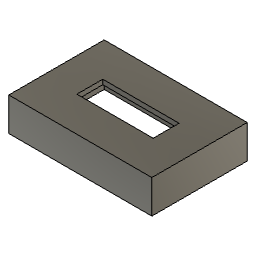
Earpiece (Autodesk Fusion 360 design; units mm, degrees)
Autodesk Fusion 360 part; units mm, degrees
sketch "Esboço1" plane through (0, 0, 0) normal (0, 0, 1) x (1, 0, 0)
  line L0 (75, 50) -> (-75, 50)
  line L1 (-75, 50) -> (-75, -50)
  line L2 (-75, -50) -> (75, -50)
  line L3 (75, -50) -> (75, 50)
  line L4 (75, 50) -> (-75, -50) construction
  line L5 (-75, 50) -> (75, -50) construction
  line L6 (-65, 40) -> (65, 40)
  line L7 (65, 40) -> (65, -40.4734)
  line L8 (65, -40.4734) -> (-65, -40.4734)
  line L9 (-65, -40.4734) -> (-65, 40)
  line L10 (39.9847, -13.5797) -> (-39.9847, -13.5797)
  line L11 (-39.9847, -13.5797) -> (-39.9847, 13.5797)
  line L12 (-39.9847, 13.5797) -> (39.9847, 13.5797)
  line L13 (39.9847, 13.5797) -> (39.9847, -13.5797)
  line L14 (39.9847, -13.5797) -> (-39.9847, 13.5797) construction
  line L15 (-39.9847, -13.5797) -> (39.9847, 13.5797) construction
  constraint horizontal L0
  constraint perpendicular L0 L1
  constraint parallel L0 L2
  constraint parallel L1 L3
  constraint coincident L4 origin
  constraint coincident L5 origin
  constraint horizontal L6
  constraint vertical L7
  constraint horizontal L8
  constraint vertical L9
  constraint horizontal L10
  constraint perpendicular L10 L11
  constraint parallel L10 L12
  constraint parallel L11 L13
  constraint coincident L14 origin
  constraint coincident L15 origin
extrude "Extrusão1" add sketch "Esboço1" along normal blind 35 contours L0 L1 L2 L3
extrude "Extrusão2" add sketch "Esboço1" along normal blind 35 contours L6 L7 L8 L9
extrude "Extrusão3" cut sketch "Esboço1" along normal blind 30 contours L6 L7 L8 L9
